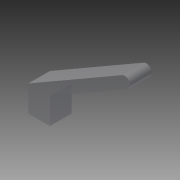
# Autodesk Inventor part: Funneling_v1
Saved by Autodesk Inventor 2013 (Build 170138000, 138)
## iProperties
Created: 2013-01-19
Part Number: Funneling_v1
Material: Polycarbonate, Clear
Document SubType Name: Modeling
Designer: motoennies
Density: 1.2 g/cm^3
Mass: 5.44846 g
Surface Area: 31.3408 cm^2
Volume: 4.54038 cm^3
Author: motoennies
Autodesk Inventor part; units mm, degrees
ref_plane "YZ Plane" through (0, 0, 0) normal (1, 0, 0) x (0, 1, 0)
ref_plane "XZ Plane" through (0, 0, 0) normal (0, 1, 0) x (-1, 0, 0)
ref_plane "XY Plane" through (0, 0, 0) normal (0, 0, 1) x (1, 0, 0)
sketch "Sketch1" plane through (0, 0, 0) normal (0, 0, 1) x (1, 0, 0)
  line L0 (0, 0) -> (0, 7.62)
  line L1 (0, 0) -> (6.35, 0)
  line L2 (0, 7.62) -> (73.3235, 7.62) construction
  line L3 (6.35, 0) -> (6.35, 7.62)
  line L4 (6.35, 7.62) -> (13.3564, 7.62) construction
  line L5 (0, 7.62) -> (60.325, 112.106)
  line L6 (6.35, 7.62) -> (65.0875, 109.3563)
  line L7 (60.325, 112.106) -> (65.0875, 109.3563)
  arc A0 (65.0875, 109.3563) -> (60.325, 112.106) centre (62.7063, 110.7311) ccw
  dimension "d0" = 7.62
  dimension "d1" = 6.35
  dimension "d8" = 7.62
  dimension "d27" = 120.65
  dimension "d28" = 60
  constraints: 16 end point, 2 horizontal, 2 perpendicular, 2 point on circle, 1 centre point, 1 midpoint, 1 parallel, 1 point on line, 1 vertical
  measures "d0" distance of L0.start L0.end
  measures "d1" distance of L0.start L1.end
  measures "d8" distance of L1.end L3.end
  measures "d27" distance of L0.end L5.end
  measures "d28" angle of L2 L5
extrude "Extrusion3" add sketch "Sketch1" along normal blind 6.35
body "Solid3"
